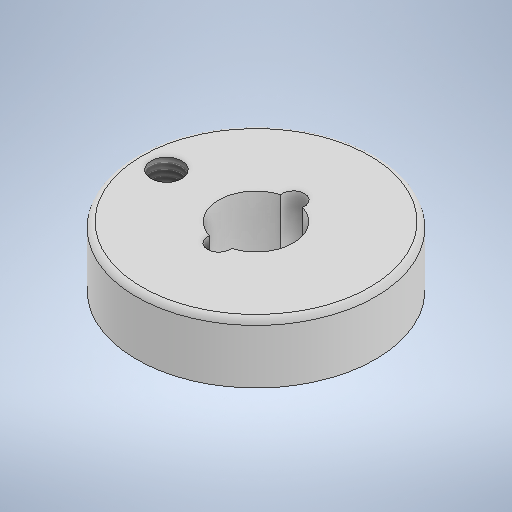
# Autodesk Inventor part: 45
Saved by Autodesk Inventor 2025.1 (Build 291241000, 241)
## iProperties
Created: 2024-09-17
Part Number: 45
Material: Generisch
Document SubType Name: Modeling
Designer: ffogue
Density: 1 g/cm^3
Appearance: Vorgabe
Author: ffogue
Autodesk Inventor part; units mm, degrees
ref_plane "YZ Plane" through (0, 0, 0) normal (1, 0, 0) x (0, 1, 0)
ref_plane "XZ Plane" through (0, 0, 0) normal (0, 1, 0) x (-1, 0, 0)
ref_plane "XY Plane" through (0, 0, 0) normal (0, 0, 1) x (1, 0, 0)
sketch "Sketch1" plane through (0, 0, 0) normal (0, 0, 1) x (1, 0, 0)
  circle A0 centre (0, 0) radius 16
  circle A1 centre (0, 0) radius 5
  dimension "d0" = 32
  dimension "d1" = 10
  constraints: 2 centre point, 2 coincident
  measures "d0" diameter of A0
  measures "d1" diameter of A1
extrude "Extrusion1" add sketch "Sketch1" along normal mid plane 8
sketch "Sketch2" plane through (0, 0, 4) normal (0, 0, 1) x (1, 0, 0)
  circle A0 centre (0, 0) radius 5 projected
  arc A1 (-1.483, -4.775) -> (1.483, -4.775) centre (0, -5) ccw
  arc A2 (1.483, 4.775) -> (-1.483, 4.775) centre (0, 5) ccw
  dimension "d4" = 3
  dimension "d5" = 3
  constraints: 10 point on circle, 2 centre point, 2 vertical alignment
  measures "d4" diameter of A1
  measures "d5" diameter of A2
extrude "Extrusion2" cut sketch "Sketch2" against normal blind 8 contours A0 A2 | A1 A0
sketch "Sketch3" plane through (0, 0, 4) normal (0, 0, 1) x (1, 0, 0)
  point P0 (0, 0)
  point P1 (-12, 0)
  dimension "d8" = 12
  constraints: 1 horizontal alignment
  measures "d8" distance of point (0, 0) point (-12, 0)
hole "Hole1" at (-12, 0, 4) direction (0, 0, -1) diameter 4.134 depth 8 thread size "M5x0.8" class "6H" standard "ISO Metric profile"
fillet "Fillet1" radius 0.75 1 edges at (-16, 0, 4)
body "Solid1"
